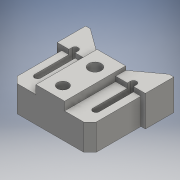
# Autodesk Inventor part: 240710_part1
Saved by Autodesk Inventor 2016 (Build 200138000, 138)
## iProperties
Created: 2024-07-10
Part Number: 240710_part1
Material: 일반
Document SubType Name: Modeling
Designer: pc
Density: 1 g/cm^3
Appearance: 기본값
Author: pc
Autodesk Inventor part; units mm, degrees
ref_plane "YZ Plane" through (0, 0, 0) normal (1, 0, 0) x (0, 1, 0)
ref_plane "XZ Plane" through (0, 0, 0) normal (0, 1, 0) x (-1, 0, 0)
ref_plane "XY Plane" through (0, 0, 0) normal (0, 0, 1) x (1, 0, 0)
sketch "스케치1" plane through (0, 0, 0) normal (0, 0, 1) x (1, 0, 0)
  line L0 (0, 11.2555) -> (-9.6591, 11.2555)
  line L1 (-9.6591, 11.2555) -> (-9.6591, -14.4887)
  line L2 (-9.6591, -14.4887) -> (0, -14.4887)
  line L3 (0, -14.4887) -> (0, 11.2555)
  point P0 (0, 0)
  constraints: 8 end point, 2 parallel, 1 horizontal, 1 perpendicular
extrude "돌출1" add sketch "스케치1" along normal blind 10
sketch "스케치2" plane through (0, 0, 10) normal (0, 0, 1) x (1, 0, 0)
  line L0 (0, 11.2555) -> (-9.6591, 11.2555) projected
  line L1 (0, -14.4887) -> (0, 11.2555) projected
  line L2 (-8.1436, 11.2555) -> (0, 5.3146)
  line L3 (0, 5.3146) -> (9.2752, 5.3146)
  line L4 (9.2752, 5.3146) -> (9.2752, -14.4887)
  line L5 (9.2752, -14.4887) -> (0, -14.4887)
  line L6 (0, -14.4887) -> (0, 5.3146)
  circle A0 centre (4.6376, 0) radius 2.0297
  circle A1 centre (4.6376, -10.4068) radius 1.7507
  line L7 (0, 2.0297) -> (-9.6591, 2.0297)
  line L8 (-9.6591, 2.0297) -> (-9.6591, -14.4887)
  line L9 (-9.6591, -14.4887) -> (0, -14.4887)
  line L10 (0, -14.4887) -> (0, 2.0297)
  arc A2 (-3.8296, 3.0291) -> (-5.8296, 3.0291) centre (-4.8296, 3.0291) ccw
  arc A3 (-5.8296, -9.1284) -> (-3.8296, -9.1284) centre (-4.8296, -9.1284) ccw
  line L11 (-5.8296, 3.0291) -> (-5.8296, -9.1284)
  line L12 (-3.8296, 3.0291) -> (-3.8296, -9.1284)
  point P0 (0, 0)
  dimension "d2" = 2
  dimension "d3" = 2
  constraints: 22 end point, 4 centre point, 4 parallel, 4 point on circle, 3 point on line, 2 horizontal, 2 perpendicular, 2 tangent
  measures "d2" diameter of A2
  measures "d3" diameter of A3
extrude "돌출2" add sketch "스케치2" against normal blind 10 contours L3 L4 L5 L1
extrude "돌출3" add sketch "스케치2" along normal blind 1.25 contours L3 L4 L5 L1
extrude "돌출4" cut sketch "스케치2" against normal up to next contours L1 L2 L0
extrude "돌출5" cut sketch "스케치2" against normal up to next contours L12 A3 L11 L7 | L7 L11 A2 L12
extrude "돌출6" cut sketch "스케치2" against normal blind 1.5 contours L1 L9 L8 L7 L11 A3 L12 | L12 A3 L11 L7
sketch "스케치3" plane through (0, 0, 8.5) normal (0, 0, 1) x (1, 0, 0)
  line L0 (0, -14.4887) -> (-9.6591, -14.4887) projected
  line L1 (-9.6591, 2.0297) -> (-8.1436, 2.0297)
  line L2 (-8.1436, 2.0297) -> (-8.1436, -14.4887)
  line L3 (-8.1436, -14.4887) -> (-9.6591, -14.4887)
  line L4 (-9.6591, -14.4887) -> (-9.6591, 2.0297)
  point P0 (0, 0)
  constraints: 8 end point, 2 parallel, 1 horizontal, 1 perpendicular, 1 point on line
extrude "돌출7" cut sketch "스케치3" against normal up to next
chamfer "모따기1" distance 2 angle 45 1 edges at (-8.1436, -14.4887, 4.25)
sketch "스케치4" plane through (0, 0, 11.25) normal (0, 0, 1) x (1, 0, 0)
  line L0 (0, -14.4887) -> (9.2752, -14.4887) projected
  line L1 (9.2752, 5.3146) -> (4.6376, 5.3146)
  line L2 (4.6376, 5.3146) -> (4.6376, -14.4887)
  line L3 (4.6376, -14.4887) -> (9.2752, -14.4887)
  line L4 (9.2752, -14.4887) -> (9.2752, 5.3146)
  point P0 (0, 0)
  constraints: 8 end point, 2 parallel, 1 horizontal, 1 midpoint, 1 perpendicular
extrude "돌출8" cut sketch "스케치4" against normal up to next
mirror "대칭1" about plane through (4.6376, -14.4887, 11.25) normal (1, 0, 0) of "돌출4", "돌출2", "돌출3", "돌출1", "돌출6", "돌출5"
sketch "스케치5" plane through (9.2752, -14.4887, 8.5) normal (0, 0, 1) x (1, 0, 0)
  line L0 (9.6591, 0) -> (0, 0) projected
  line L1 (9.6591, 16.5185) -> (8.2337, 16.5185)
  line L2 (8.2337, 16.5185) -> (8.2337, 0)
  line L3 (8.2337, 0) -> (9.6591, 0)
  line L4 (9.6591, 0) -> (9.6591, 16.5185)
  point P0 (-9.2752, 14.4887)
  constraints: 8 end point, 2 parallel, 1 horizontal, 1 perpendicular, 1 point on line
extrude "돌출9" cut sketch "스케치5" against normal up to next
chamfer "모따기2" distance 2 angle 45 1 edges at (17.5089, -14.4887, 4.25)
